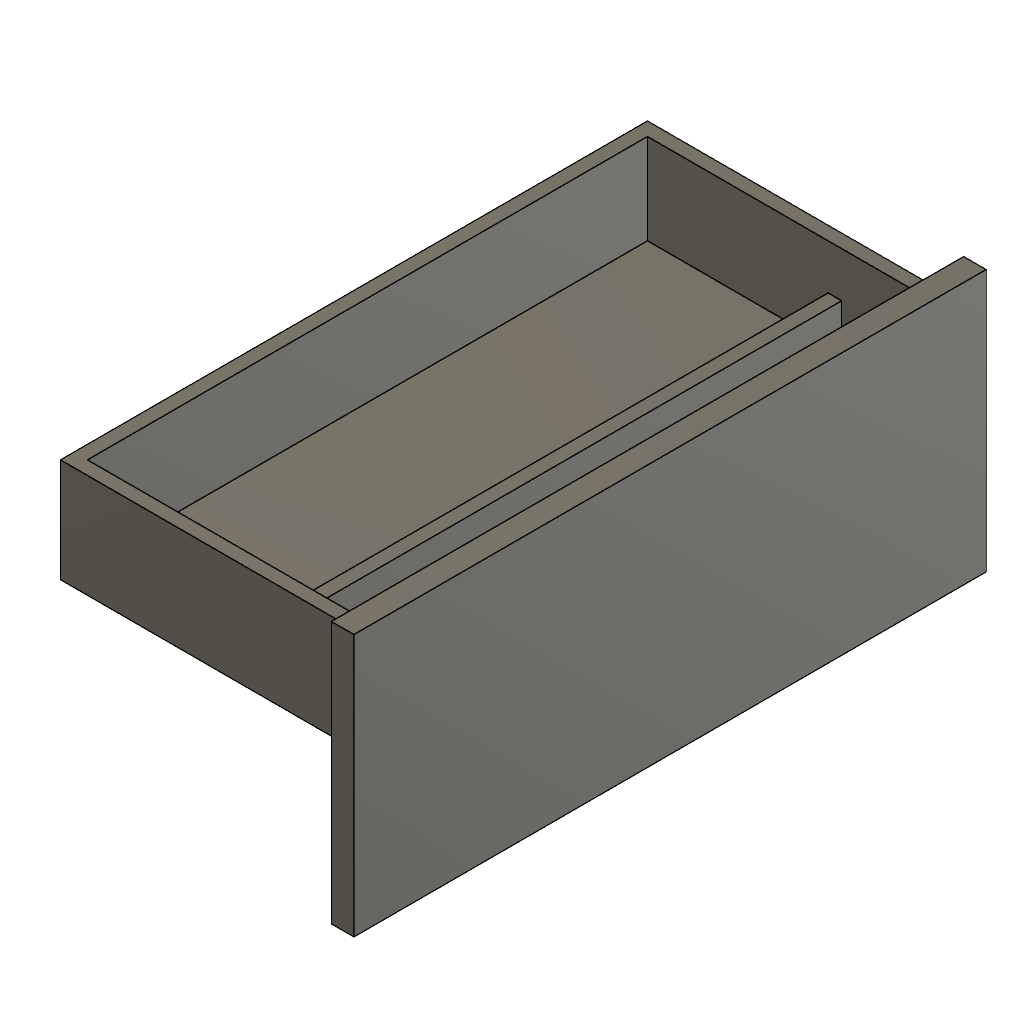
BALANCIN_V2 (Autodesk Fusion 360 archive; units mm, degrees)
design "CAJA BATERIA"
part number: 2026-09-12-01-05-41-271
Autodesk Fusion 360 part; units mm, degrees
sketch "Boceto9" plane through (0, 0, 0) normal (1, 0, 0) x (0, 0, -1)
  line L0 (0, 0) -> (130, 0)
  line L1 (130, 0) -> (130, 3)
  line L2 (130, 3) -> (0, 3)
  line L3 (0, 3) -> (0, 0)
  dimension "d48" = 130
  dimension "d49" = 3
  constraint horizontal L0
  constraint vertical L1
  constraint horizontal L2
  constraint vertical L3
  constraint coincident L0.start L3.end
  measures "d48" distance of L0.start L0.end
  measures "d49" distance of L0.start L2.end
extrude "Extruir9" add sketch "Boceto9" against normal blind 65
sketch "Boceto10" plane through (0, 0, 0) normal (1, 0, 0) x (0, 0, -1)
  line L0 (0, 0) -> (-5, 0)
  line L1 (-5, 0) -> (-5, 27)
  line L2 (-5, 27) -> (135, 27)
  line L3 (135, 27) -> (135, -31)
  line L4 (135, -31) -> (-5, -31)
  line L5 (-5, -31) -> (-5, 27)
  dimension "d64" = 5
  dimension "d65" = 27
  dimension "d66" = 140
  dimension "d67" = 58
  constraint coincident L0.start origin
  constraint horizontal L0
  constraint perpendicular L0 L1
  constraint horizontal L2
  constraint vertical L3
  constraint horizontal L4
  constraint vertical L5
  measures "d64" distance of L0.start L0.end
  measures "d65" distance of L0.end L1.end
  measures "d66" distance of L1.end L2.end
  measures "d67" distance of L1.end L4.end
extrude "Extruir10" add sketch "Boceto10" along normal blind 5
sketch "Boceto11" plane through (0, 3, 0) normal (0, 1, 0) x (-1, 0, 0)
  line L0 (0, 0) -> (0, -130)
  line L1 (0, -130) -> (65, -130)
  line L2 (65, -130) -> (65, 0)
  line L3 (65, 0) -> (0, 0)
  line L4 (0, -130) -> (65, -130)
  line L5 (65, -130) -> (65, -127)
  line L6 (65, -127) -> (0, -127)
  line L7 (0, -127) -> (0, -130)
  line L8 (65, -130) -> (62, -130)
  line L9 (62, -130) -> (62, 0)
  line L10 (62, 0) -> (65, 0)
  line L11 (65, 0) -> (65, -130)
  line L12 (0, 0) -> (65, 0)
  line L13 (65, 0) -> (65, -3)
  line L14 (65, -3) -> (0, -3)
  line L15 (0, -3) -> (0, 0)
  dimension "d59" = 3
  dimension "d60" = 3
  dimension "d61" = 3
  constraint horizontal L4
  constraint vertical L5
  constraint horizontal L6
  constraint vertical L7
  constraint coincident L0.end L1.start
  constraint horizontal L8
  constraint vertical L9
  constraint horizontal L10
  constraint vertical L11
  constraint horizontal L12
  constraint vertical L13
  constraint horizontal L14
  constraint vertical L15
  constraint coincident L0.start L3.end
  measures "d59" distance of L0.end L6.end
  measures "d60" distance of L1.end L8.end
  measures "d61" distance of L0.start L14.end
extrude "Extruir11" add sketch "Boceto11" along normal blind 20 contours L0 L3 L9 L12 L14 L15 | L2 L3 L9 L10 L11 L12 L13 L14 | L0 L1 L4 L6 L7 L9 | L2 L6 L9 L11 L14 | L1 L2 L4 L5 L6 L8 L9 L11
sketch "Boceto12" plane through (0, 3, 0) normal (0, 1, 0) x (-1, 0, 0)
  line L0 (62, -3) -> (0, -3)
  line L1 (0, -3) -> (0, -127)
  line L2 (0, -127) -> (62, -127)
  line L3 (62, -127) -> (62, -3)
  line L4 (62, -127) -> (22, -127)
  line L5 (22, -127) -> (19, -127)
  line L6 (19, -127) -> (19, -7)
  line L7 (19, -7) -> (22, -7)
  line L8 (22, -7) -> (22, -127)
  line L9 (19, -7) -> (39, -7)
  line L10 (39, -7) -> (39, -3)
  line L11 (39, -3) -> (19, -3)
  line L12 (19, -3) -> (19, -7)
  dimension "d68" = 40
  dimension "d69" = 3
  dimension "d70" = 120
  dimension "d71" = 20
  constraint coincident L2.end L3.start
  constraint perpendicular L3 L4
  constraint horizontal L5
  constraint vertical L6
  constraint horizontal L7
  constraint vertical L8
  constraint horizontal L9
  constraint vertical L10
  constraint horizontal L11
  constraint vertical L12
  measures "d68" distance of L2.end L4.end
  measures "d69" distance of L4.end L5.end
  measures "d70" distance of L4.end L7.end
  measures "d71" distance of L6.end L9.end
extrude "Extruir12" add sketch "Boceto12" along normal blind 10 contours L0 L7 L9 L10 L11 L12 | L2 L5 L6 L7 L8 L9

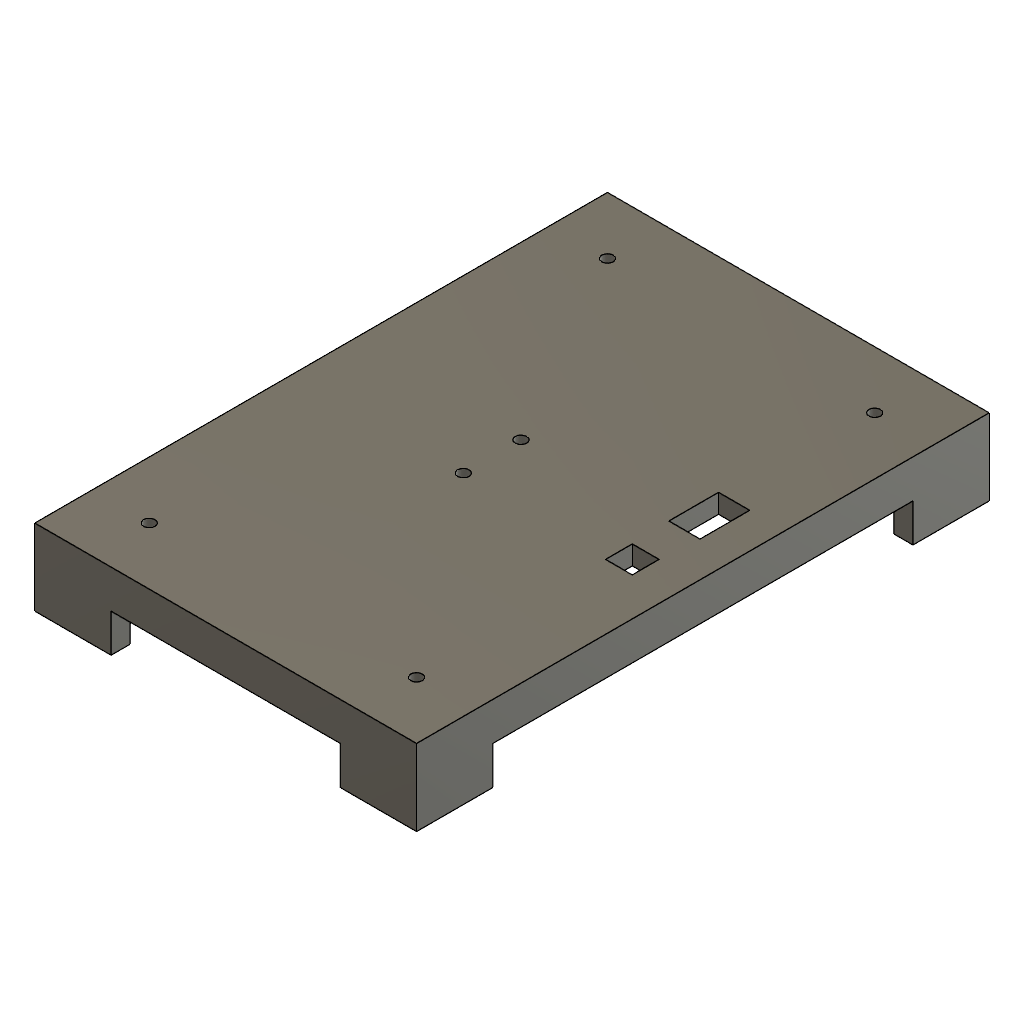
design "TAPA"
part number: 2026-09-12-01-46-28-572
Autodesk Fusion 360 part; units mm, degrees
sketch "Boceto11" plane through (0, 0, 0) normal (0, 1, 0) x (1, 0, 0)
  line L0 (0, 0) -> (100, 0)
  line L1 (100, 0) -> (100, -150)
  line L2 (100, -150) -> (0, -150)
  line L3 (0, -150) -> (0, 0)
  dimension "d80" = 100
  dimension "d81" = 150
  constraint horizontal L0
  constraint vertical L1
  constraint horizontal L2
  constraint vertical L3
  constraint coincident L0.start L3.end
  measures "d80" distance of L0.start L0.end
  measures "d81" distance of L0.start L2.end
extrude "Extruir1" add sketch "Boceto11" along normal blind 5 from surface at 15
sketch "Boceto3" plane through (0, 15, 0) normal (0, -1, 0) x (1, 0, 0)
  line L0 (0, 0) -> (100, 0)
  line L1 (100, 0) -> (100, 5)
  line L2 (100, 5) -> (0, 5)
  line L3 (0, 5) -> (0, 0)
  line L4 (100, 0) -> (95, 0)
  line L5 (95, 0) -> (95, 150)
  line L6 (95, 150) -> (100, 150)
  line L7 (100, 150) -> (100, 0)
  line L8 (100, 150) -> (0, 150)
  line L9 (0, 150) -> (0, 145)
  line L10 (0, 145) -> (100, 145)
  line L11 (100, 145) -> (100, 150)
  line L12 (0, 150) -> (5, 150)
  line L13 (5, 150) -> (5, 0)
  line L14 (5, 0) -> (0, 0)
  line L15 (0, 0) -> (0, 150)
  dimension "d155" = 5
  dimension "d156" = 5
  dimension "d157" = 150
  dimension "d158" = 100
  dimension "d159" = 5
  dimension "d160" = 5
  dimension "d161" = 150
  constraint horizontal L0
  constraint vertical L1
  constraint horizontal L2
  constraint vertical L3
  constraint coincident L0.start L3.end
  constraint horizontal L4
  constraint vertical L5
  constraint horizontal L6
  constraint vertical L7
  constraint horizontal L8
  constraint vertical L9
  constraint horizontal L10
  constraint vertical L11
  constraint horizontal L12
  constraint vertical L13
  constraint horizontal L14
  constraint vertical L15
  measures "d155" distance of L0.start L2.end
  measures "d156" distance of L0.end L4.end
  measures "d157" distance of L0.end L6.end
  measures "d158" distance of L6.end L8.end
  measures "d159" distance of L6.end L10.end
  measures "d160" distance of L8.end L12.end
  measures "d161" distance of L8.end L0.start
extrude "Extruir2" add sketch "Boceto3" along normal blind 15 contours L0 L2 L3 L13 L14 L15 | L0 L2 L5 L13 | L2 L10 L13 L15 | L0 L1 L2 L4 L5 L7 | L8 L9 L10 L12 L13 L15 | L2 L5 L7 L10 | L5 L8 L10 L13 | L5 L6 L7 L8 L10 L11
sketch "Boceto14" plane through (0, 20, 0) normal (0, 1, 0) x (-1, 0, 0)
  line L0 (0, 150) -> (-100, 150)
  line L1 (-100, 150) -> (-100, 0)
  line L2 (-100, 0) -> (0, 0)
  line L3 (0, 0) -> (0, 150)
  line L4 (-100, 150) -> (-100, 80)
  line L5 (-100, 80) -> (-90, 80)
  line L6 (-90, 80) -> (-90, 76.5)
  line L7 (-90, 76.5) -> (-83, 76.5)
  line L8 (-83, 76.5) -> (-83, 83.5)
  line L9 (-83, 83.5) -> (-90, 83.5)
  line L10 (-90, 83.5) -> (-90, 76.5)
  line L11 (-86.5, 76.5) -> (-86.5, 66.5)
  line L12 (-86.5, 66.5) -> (-100, 66.5)
  line L13 (-86.5, 66.5) -> (-82.5879, 66.5)
  line L14 (-82.5879, 66.5) -> (-90.7379, 66.5)
  line L15 (-90.7379, 66.5) -> (-90.7379, 53.5)
  line L16 (-90.7379, 53.5) -> (-82.5879, 53.5)
  line L17 (-82.5879, 53.5) -> (-82.5879, 66.5)
  dimension "d106" = 70
  dimension "d107" = 10
  dimension "d108" = 3.5
  dimension "d109" = 7
  dimension "d110" = 7
  dimension "d122" = 10
  dimension "d123" = 8.15
  dimension "d124" = 13
  constraint coincident L0.end L1.start
  constraint perpendicular L0 L4
  constraint perpendicular L4 L5
  constraint perpendicular L5 L6
  constraint horizontal L7
  constraint vertical L8
  constraint horizontal L9
  constraint vertical L10
  constraint midpoint L7 L11.start
  constraint perpendicular L7 L11
  constraint coincident L1 L12.end
  constraint perpendicular L1 L12
  constraint perpendicular L11 L13
  constraint horizontal L14
  constraint vertical L15
  constraint horizontal L16
  constraint vertical L17
  measures "d106" distance of L0.end L4.end
  measures "d107" distance of L4.end L5.end
  measures "d108" distance of L5.end L6.end
  measures "d109" distance of L6.end L7.end
  measures "d110" distance of L6.end L9.end
  measures "d122" distance of L11.start L11.end
  measures "d123" distance of L13.end L14.end
  measures "d124" distance of L13.end L16.end
extrude "Extruir9" cut sketch "Boceto14" against normal blind 30 contours L6 L7 L8 L9 L10 | L12 L13 L14 L15 L16 L17
sketch "Boceto15" plane through (0, 0, 150) normal (0, 0, 1) x (1, 0, 0)
  line L0 (100, 0) -> (100, 20)
  line L1 (100, 20) -> (0, 20)
  line L2 (0, 20) -> (0, 0)
  line L3 (0, 0) -> (100, 0)
  line L4 (0, 0) -> (20, 0)
  line L5 (100, 0) -> (80, 0)
  line L6 (80, 0) -> (20, 0)
  line L7 (20, 0) -> (20, 10)
  line L8 (20, 10) -> (80, 10)
  line L9 (80, 10) -> (80, 0)
  dimension "d113" = 20
  dimension "d114" = 20
  dimension "d115" = 10
  constraint coincident L2.end L3.start
  constraint perpendicular L2 L4
  constraint coincident L0.start L3.end
  constraint perpendicular L0 L5
  constraint horizontal L6
  constraint vertical L7
  constraint horizontal L8
  constraint vertical L9
  measures "d113" distance of L2.end L4.end
  measures "d114" distance of L0.start L5.end
  measures "d115" distance of L5.end L8.end
extrude "Extruir10" cut sketch "Boceto15" against normal blind 180 contours L3 L6 L7 L8 L9
sketch "Boceto16" plane through (100, 0, 0) normal (1, 0, 0) x (0, 0, -1)
  line L0 (0, 0) -> (0, 20)
  line L1 (0, 20) -> (-150, 20)
  line L2 (-150, 20) -> (-150, 0)
  line L3 (-150, 0) -> (0, 0)
  line L4 (0, 0) -> (-20, 0)
  line L5 (-150, 0) -> (-130, 0)
  line L6 (-130, 0) -> (-20, 0)
  line L7 (-20, 0) -> (-20, 10)
  line L8 (-20, 10) -> (-130, 10)
  line L9 (-130, 10) -> (-130, 0)
  dimension "d118" = 20
  dimension "d119" = 20
  constraint coincident L0.start L3.end
  constraint perpendicular L0 L4
  constraint coincident L2.end L3.start
  constraint perpendicular L2 L5
  constraint horizontal L6
  constraint vertical L7
  constraint horizontal L8
  constraint vertical L9
  measures "d118" distance of L0.start L4.end
  measures "d119" distance of L2.end L5.end
extrude "Extruir11" cut sketch "Boceto16" against normal blind 130 contours L3 L6 L7 L8 L9
sketch "Boceto17" plane through (0, 20, 0) normal (0, 1, 0) x (-1, 0, 0)
  line L0 (-83, 76.5) -> (-90, 76.5)
  line L1 (-90, 76.5) -> (-90, 83.5)
  line L2 (-90, 83.5) -> (-83, 83.5)
  line L3 (-83, 83.5) -> (-83, 76.5)
  line L4 (-90.7379, 66.5) -> (-82.5879, 66.5)
  line L5 (-82.5879, 66.5) -> (-82.5879, 53.5)
  line L6 (-82.5879, 53.5) -> (-90.7379, 53.5)
  line L7 (-90.7379, 53.5) -> (-90.7379, 66.5)
  line L8 (0, 150) -> (-100, 150)
  line L9 (-100, 150) -> (-100, 0)
  line L10 (-100, 0) -> (0, 0)
  line L11 (0, 0) -> (0, 150)
  line L12 (-100, 0) -> (-85, 0)
  line L13 (-85, 0) -> (-85, 15)
  circle A0 centre (-85, 15) radius 1.5
  line L14 (0, 0) -> (-15, 0)
  line L15 (-15, 0) -> (-15, 15)
  circle A1 centre (-15, 15) radius 1.5
  line L16 (0, 150) -> (-15, 150)
  line L17 (-15, 150) -> (-15, 135)
  circle A2 centre (-15, 135) radius 1.5
  line L18 (-100, 150) -> (-85, 150)
  line L19 (-85, 150) -> (-85, 135)
  circle A3 centre (-85, 135) radius 1.5
  dimension "d125" = 15
  dimension "d126" = 15
  dimension "d127" = 3
  dimension "d128" = 15
  dimension "d129" = 15
  dimension "d130" = 3
  dimension "d131" = 15
  dimension "d132" = 15
  dimension "d133" = 3
  dimension "d134" = 15
  dimension "d135" = 15
  dimension "d136" = 3
  constraint coincident L9.end L10.start
  constraint perpendicular L9 L12
  constraint perpendicular L10 L13
  constraint coincident L13.end A0.centre
  constraint coincident L10.end L11.start
  constraint perpendicular L11 L14
  constraint perpendicular L10 L15
  constraint coincident L15.end A1.centre
  constraint coincident L8.start L11.end
  constraint perpendicular L11 L16
  constraint perpendicular L8 L17
  constraint coincident L17.end A2.centre
  constraint coincident L8.end L9.start
  constraint perpendicular L9 L18
  constraint perpendicular L8 L19
  constraint coincident L19.end A3.centre
  measures "d125" distance of L9.end L12.end
  measures "d126" distance of L12.end L13.end
  measures "d127" diameter of A0
  measures "d128" distance of L10.end L14.end
  measures "d129" distance of L14.end L15.end
  measures "d130" diameter of A1
  measures "d131" distance of L8.start L16.end
  measures "d132" distance of L16.end L17.end
  measures "d133" diameter of A2
  measures "d134" distance of L8.end L18.end
  measures "d135" distance of L18.end L19.end
  measures "d136" diameter of A3
extrude "Extruir12" cut sketch "Boceto17" against normal blind 20 contours A0 | A1 | A2 | A3
sketch "Boceto18" plane through (0, 15, 0) normal (0, -1, 0) x (1, 0, 0)
  line L0 (95, 140) -> (95, 10)
  line L1 (95, 140) -> (95, 75)
  line L2 (95, 75) -> (50, 75)
  line L3 (50, 75) -> (50, 85.35)
  line L4 (50, 85.35) -> (42, 85.35)
  line L5 (42, 85.35) -> (58, 85.35)
  line L6 (58, 85.35) -> (58, 64.65)
  line L7 (58, 64.65) -> (42, 64.65)
  line L8 (42, 64.65) -> (42, 85.35)
  line L9 (95, 145) -> (5, 145)
  line L10 (5, 145) -> (5, 5)
  line L11 (5, 5) -> (95, 5)
  line L12 (95, 5) -> (95, 145)
  line L13 (82.5879, 66.5) -> (90.7379, 66.5)
  line L14 (90.7379, 66.5) -> (90.7379, 53.5)
  line L15 (90.7379, 53.5) -> (82.5879, 53.5)
  line L16 (82.5879, 53.5) -> (82.5879, 66.5)
  line L17 (90, 76.5) -> (83, 76.5)
  line L18 (83, 76.5) -> (83, 83.5)
  line L19 (83, 83.5) -> (90, 83.5)
  line L20 (90, 83.5) -> (90, 76.5)
  circle A0 centre (15, 135) radius 1.5
  circle A1 centre (15, 15) radius 1.5
  circle A2 centre (85, 135) radius 1.5
  circle A3 centre (85, 15) radius 1.5
  line L21 (100, 0) -> (0, 0)
  dimension "d140" = 45
  dimension "d141" = 10.35
  dimension "d142" = 8
  dimension "d143" = 16
  dimension "d144" = 20.7
  dimension "d162" = 75
  constraint midpoint L0 L1.end
  constraint perpendicular L2 L3
  constraint perpendicular L3 L4
  constraint horizontal L5
  constraint vertical L6
  constraint horizontal L7
  constraint vertical L8
  measures "d140" distance of L1.end L2.end
  measures "d141" distance of L2.end L3.end
  measures "d142" distance of L3.end L4.end
  measures "d143" distance of L4.end L5.end
  measures "d144" distance of L4.end L7.end
  measures "d162" distance of L2 L21
extrude "Extruir13" cut sketch "Boceto18" against normal blind 2 contours L2 L3 L4 L5 L6 L7 L8 | L2 L3 L5 L6
sketch "Boceto19" plane through (0, 17, 0) normal (0, -1, 0) x (1, 0, 0)
  line L0 (42, 64.65) -> (58, 64.65)
  line L1 (58, 64.65) -> (58, 85.35)
  line L2 (58, 85.35) -> (42, 85.35)
  line L3 (42, 85.35) -> (42, 64.65)
  line L4 (42, 64.65) -> (44.8, 64.65)
  line L5 (44.8, 64.65) -> (44.8, 67.45)
  line L6 (44.8, 67.45) -> (42, 67.45)
  line L7 (42, 67.45) -> (42, 64.65)
  line L8 (42, 85.35) -> (44.8, 85.35)
  line L9 (44.8, 85.35) -> (44.8, 82.55)
  line L10 (44.8, 82.55) -> (42, 82.55)
  line L11 (42, 82.55) -> (42, 85.35)
  circle A0 centre (44.8, 82.55) radius 1.5
  circle A1 centre (44.8, 67.45) radius 1.5
  dimension "d147" = 2.8
  dimension "d148" = 2.8
  dimension "d149" = 2.8
  dimension "d150" = 2.8
  dimension "d163" = 20.7
  dimension "d164" = 16
  dimension "d165" = 3
  dimension "d166" = 3
  constraint horizontal L4
  constraint vertical L5
  constraint horizontal L6
  constraint vertical L7
  constraint coincident L0.start L3.end
  constraint horizontal L8
  constraint vertical L9
  constraint horizontal L10
  constraint vertical L11
  constraint coincident L2.end L3.start
  constraint coincident L9.end L10.start
  constraint coincident L5.end L6.start
  measures "d147" distance of L0.start L4.end
  measures "d148" distance of L0.start L6.end
  measures "d149" distance of L2.end L8.end
  measures "d150" distance of L2.end L10.end
  measures "d163" distance of L0 L2
  measures "d164" distance of L1 L3
  measures "d165" diameter of A0
  measures "d166" diameter of A1
extrude "Extruir14" cut sketch "Boceto19" against normal blind 3.5 contours L5 L6 A1 | L5 L6 A1 | L9 L10 A0 | L9 L10 A0

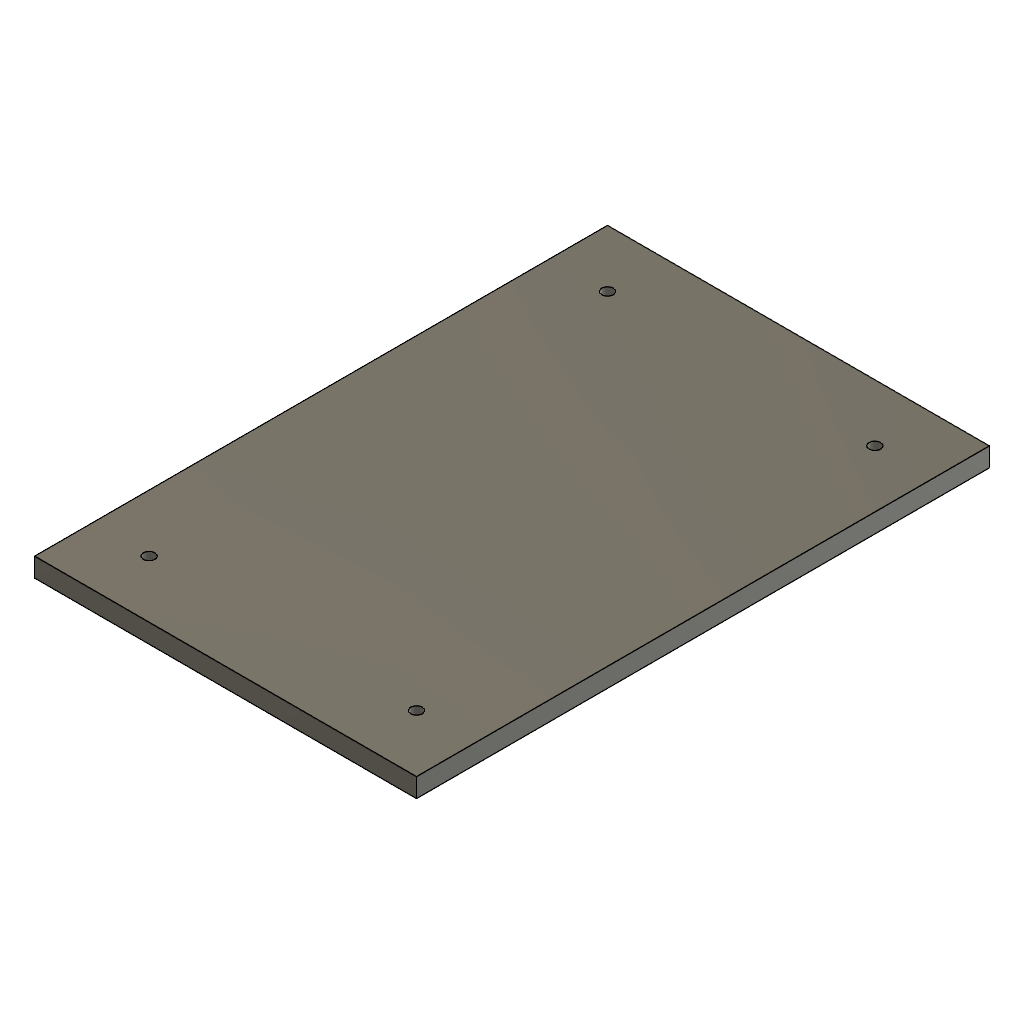
design "PLACA"
part number: 2026-09-12-02-16-54-781
Autodesk Fusion 360 part; units mm, degrees
sketch "Boceto1" plane through (2.5309, 197.6555, 0.0134) normal (0, 1, 0) x (-1, 0, 0)
  line L0 (0, 0) -> (-100, 0)
  line L1 (-100, 0) -> (-100, 150)
  line L2 (-100, 150) -> (0, 150)
  line L3 (0, 150) -> (0, 0)
  line L4 (-100, 150) -> (-85, 150)
  line L5 (-85, 150) -> (-85, 135)
  line L6 (0, 150) -> (-15, 150)
  line L7 (-15, 150) -> (-15, 135)
  line L8 (-100, 0) -> (-85, 0)
  line L9 (-85, 0) -> (-85, 15)
  line L10 (0, 0) -> (-15, 0)
  line L11 (-15, 0) -> (-15, 15)
  circle A0 centre (-15, 15) radius 1.5
  circle A1 centre (-85, 15) radius 1.5
  circle A2 centre (-15, 135) radius 1.5
  circle A3 centre (-85, 135) radius 1.5
  dimension "d3" = 100
  dimension "d4" = 150
  dimension "d5" = 15
  dimension "d6" = 15
  dimension "d7" = 15
  dimension "d8" = 15
  dimension "d9" = 15
  dimension "d10" = 15
  dimension "d11" = 15
  dimension "d12" = 3
  dimension "d13" = 3
  dimension "d14" = 3
  dimension "d15" = 3
  dimension "d16" = 15
  constraint horizontal L0
  constraint vertical L1
  constraint horizontal L2
  constraint vertical L3
  constraint coincident L0.start L3.end
  constraint perpendicular L1 L4
  constraint perpendicular L2 L5
  constraint perpendicular L3 L6
  constraint perpendicular L2 L7
  constraint perpendicular L1 L8
  constraint perpendicular L8 L9
  constraint coincident L0 L10.end
  constraint perpendicular L0 L11
  constraint coincident L11.end A0.centre
  constraint coincident L9.end A1.centre
  constraint coincident L7.end A2.centre
  constraint coincident L5.end A3.centre
  measures "d3" distance of L0.start L0.end
  measures "d4" distance of L0.start L2.end
  measures "d5" distance of L1.end L4.end
  measures "d6" distance of L4.end L5.end
  measures "d7" distance of L2.end L6.end
  measures "d8" distance of L6.end L7.end
  measures "d9" distance of L0.end L8.end
  measures "d10" distance of L8.end L9.end
  measures "d11" distance of L0.start L10.end
  measures "d12" diameter of A0
  measures "d13" diameter of A1
  measures "d14" diameter of A2
  measures "d15" diameter of A3
  measures "d16" distance of L10.end L11.end
extrude "Extruir1" add sketch "Boceto1" along normal blind 5

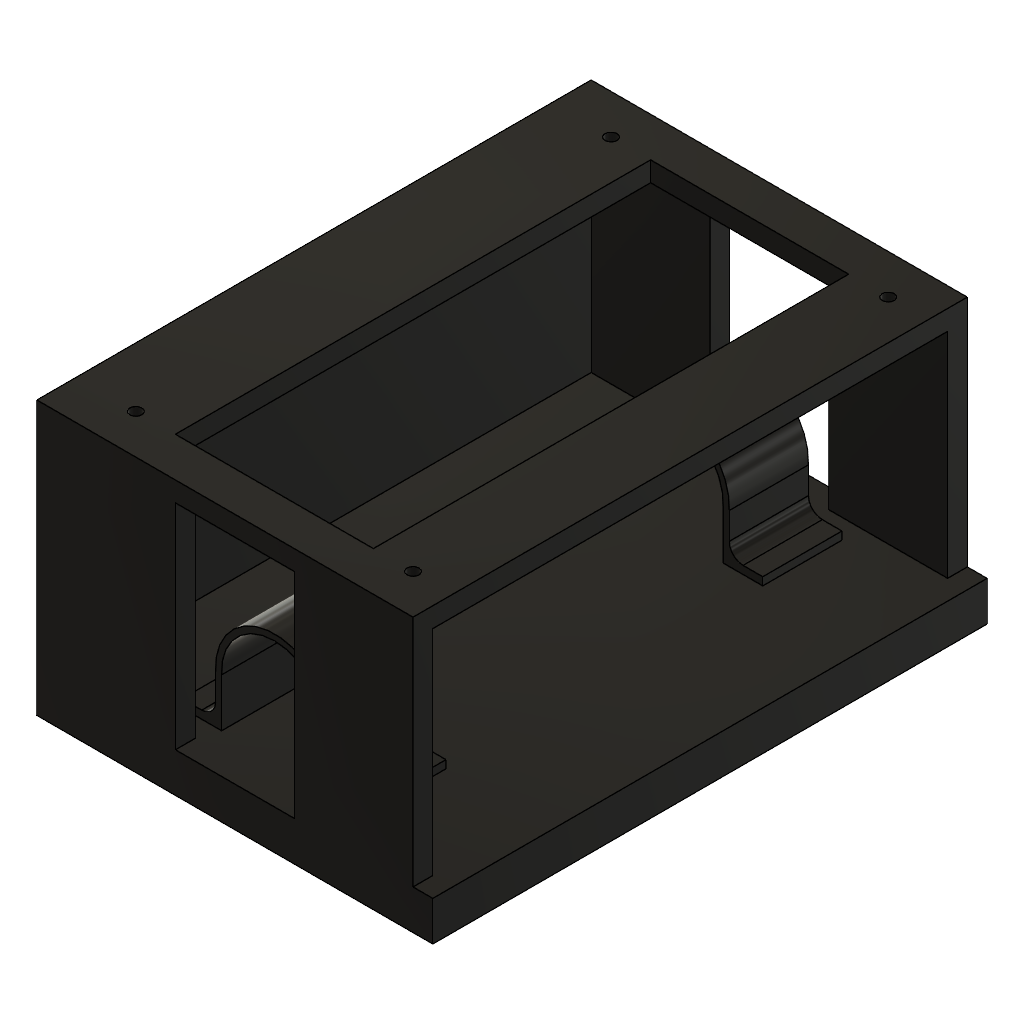
design "BASE"
part number: 2026-09-12-00-28-25-812
Autodesk Fusion 360 part; units mm, degrees
other "DerivedContext1"
sketch "Boceto3" plane through (0, 0, 0) normal (1, 0, 0) x (0, 0, -1)
  line L0 (0, 0) -> (0, 20)
  line L1 (0, 20) -> (-70, 20)
  line L2 (0, 20) -> (70, 20)
  line L3 (-70, 20) -> (70, 20)
  line L4 (70, 20) -> (70, 10)
  line L5 (70, 10) -> (-70, 10)
  line L6 (-70, 10) -> (-70, 20)
  dimension "d3" = 10
  dimension "d17" = 20
  dimension "d75" = 70
  dimension "d76" = 70
  constraint coincident L0.start origin
  constraint perpendicular L0 L1
  constraint perpendicular L0 L2
  constraint horizontal L3
  constraint vertical L4
  constraint horizontal L5
  constraint vertical L6
  measures "d3" distance of L1.end L5.end
  measures "d17" distance of L0.start L0.end
  measures "d75" distance of L0 L4
  measures "d76" distance of L0 L6
extrude "Extruir1" add sketch "Boceto3" along normal mid plane 100
sketch "Boceto4" plane through (0, 20, 0) normal (0, 1, 0) x (-1, 0, 0)
  line L0 (-50, 70) -> (50, 70)
  line L1 (50, 70) -> (50, 65)
  line L2 (50, 65) -> (-50, 65)
  line L3 (-50, 65) -> (-50, 70)
  line L4 (50, -70) -> (-50, -70)
  line L5 (-50, -70) -> (-50, -65)
  line L6 (-50, -65) -> (50, -65)
  line L7 (50, -65) -> (50, -70)
  line L8 (50, 70) -> (45, 70)
  line L9 (45, 70) -> (45, -70)
  line L10 (45, -70) -> (50, -70)
  line L11 (50, -70) -> (50, 70)
  line L12 (-50, 70) -> (0, 70)
  line L13 (0, 70) -> (-15, 70)
  line L14 (-15, 70) -> (-15, 65)
  line L15 (-15, 65) -> (0, 65)
  line L16 (0, 70) -> (15, 70)
  line L17 (15, 70) -> (15, 65)
  line L18 (15, 65) -> (0, 65)
  line L19 (0, -65) -> (-15, -65)
  line L20 (-15, -65) -> (-15, -70)
  line L21 (-15, -70) -> (0, -70)
  line L22 (0, -65) -> (15, -65)
  line L23 (15, -65) -> (15, -70)
  line L24 (15, -70) -> (0, -70)
  line L25 (-50, -70) -> (-45, -70)
  line L26 (-45, -70) -> (-45, -65)
  line L27 (-45, -65) -> (-50, -65)
  line L28 (-50, -65) -> (-50, -70)
  line L29 (-50, 70) -> (-45, 70)
  line L30 (-45, 70) -> (-45, 65)
  line L31 (-45, 65) -> (-50, 65)
  line L32 (-50, 65) -> (-50, 70)
  dimension "d77" = 100
  dimension "d78" = 5
  dimension "d83" = 15
  dimension "d84" = 15
  dimension "d85" = 15
  dimension "d86" = 5
  dimension "d87" = 15
  dimension "d88" = 5
  dimension "d97" = 5
  dimension "d98" = 5
  dimension "d99" = 5
  constraint horizontal L0
  constraint vertical L1
  constraint horizontal L2
  constraint vertical L3
  constraint horizontal L4
  constraint vertical L5
  constraint horizontal L6
  constraint vertical L7
  constraint horizontal L8
  constraint vertical L9
  constraint horizontal L10
  constraint vertical L11
  constraint coincident L4 L9.end
  constraint midpoint L0 L12.end
  constraint horizontal L13
  constraint vertical L14
  constraint horizontal L15
  constraint horizontal L16
  constraint vertical L17
  constraint horizontal L18
  constraint horizontal L19
  constraint vertical L20
  constraint horizontal L21
  constraint midpoint L6 L19.start
  constraint horizontal L22
  constraint vertical L23
  constraint horizontal L24
  constraint horizontal L25
  constraint vertical L26
  constraint horizontal L27
  constraint vertical L28
  constraint horizontal L29
  constraint vertical L30
  constraint horizontal L31
  constraint vertical L32
  measures "d77" distance of L0.start L0.end
  measures "d78" distance of L0.start L2.end
  measures "d83" distance of L12.end L13.end
  measures "d84" distance of L12.end L16.end
  measures "d85" distance of L19.start L19.end
  measures "d86" distance of L19.start L21.end
  measures "d87" distance of L19.start L22.end
  measures "d88" distance of L19.start L21.end
  measures "d97" distance of L4.end L25.end
  measures "d98" distance of L0.start L29.end
  measures "d99" distance of L0.start L2.end
extrude "Extruir2" add sketch "Boceto4" along normal blind 54 contours L0 L2 L12 L14 L30 | L0 L2 L9 L17 | L0 L1 L2 L8 L9 L11 | L2 L6 L9 L11 | L4 L6 L9 L23 | L4 L6 L7 L9 L10 L11 | L4 L6 L20 L26
sketch "Boceto6" plane through (0, 74, 0) normal (0, 1, 0) x (-1, 0, 0)
  line L0 (50, -70) -> (25, -70)
  line L1 (25, -70) -> (25, 70)
  line L2 (25, 70) -> (50, 70)
  line L3 (50, 70) -> (50, -70)
  line L4 (25, -70) -> (-25, -70)
  line L5 (-25, -70) -> (-25, -60)
  line L6 (-25, -60) -> (25, -60)
  line L7 (25, -60) -> (25, -70)
  line L8 (-50, -70) -> (-25, -70)
  line L9 (-25, -70) -> (-25, 70)
  line L10 (25, 60) -> (25, 70)
  line L11 (25, 70) -> (-25, 70)
  line L12 (-25, 70) -> (-25, 60)
  line L13 (-25, 60) -> (25, 60)
  line L14 (25, 60) -> (25, 70)
  line L15 (-45, -70) -> (-25, -70)
  line L16 (-25, -70) -> (-25, 70)
  line L17 (-25, 70) -> (-45, 70)
  line L18 (-45, 70) -> (-45, -70)
  dimension "d89" = 25
  dimension "d90" = 50
  dimension "d91" = 10
  dimension "d95" = 25
  dimension "d96" = 10
  constraint horizontal L0
  constraint vertical L1
  constraint horizontal L2
  constraint vertical L3
  constraint horizontal L4
  constraint vertical L5
  constraint horizontal L6
  constraint vertical L7
  constraint horizontal L8
  constraint vertical L9
  constraint vertical L10
  constraint horizontal L11
  constraint vertical L12
  constraint horizontal L13
  constraint vertical L14
  constraint horizontal L15
  constraint vertical L16
  constraint horizontal L17
  constraint vertical L18
  constraint coincident L8 L15.start
  measures "d89" distance of L0.start L0.end
  measures "d90" distance of L0.end L4.end
  measures "d91" distance of L0.end L6.end
  measures "d95" distance of L8.start L4.end
  measures "d96" distance of L1.end L10.start
extrude "Extruir4" add sketch "Boceto6" 1 faces at (-48.3333, 74, -21.6667) along normal blind 5 contours L0 L1 L2 L3 L7 L10 L14 | L1 L4 L5 L6 L7 L9 L16 | L5 L8 L9 L12 L15 L16 L17 L18 | L1 L9 L10 L11 L12 L13 L14 L16
sketch "Boceto8" plane through (0, 0, 0) normal (0, 0, 1) x (1, 0, 0)
  circle A0 centre (0, 33) radius 13.3417
  circle A1 centre (0, 33) radius 14.8661
  line L0 (-14.8465, 32.2379) -> (-14.8465, 25.5)
  line L1 (-13.3199, 32.2379) -> (-13.3199, 20)
  line L2 (14.8465, 32.2379) -> (14.8465, 25.5)
  line L3 (13.3199, 32.2379) -> (13.3199, 20)
  line L4 (13.3199, 20) -> (14.8465, 20)
  line L5 (-14.8465, 20) -> (-13.3199, 20)
  line L6 (-13.3199, 20) -> (-23.3199, 20)
  line L7 (-23.3199, 20) -> (-23.3199, 22)
  line L8 (-23.3199, 22) -> (-18.3465, 22)
  line L9 (-13.3199, 22) -> (-13.3199, 20)
  arc A2 (-18.3465, 22) -> (-14.8465, 25.5) centre (-18.3465, 25.5) ccw
  line L10 (13.3199, 20) -> (23.3199, 20)
  line L11 (23.3199, 20) -> (23.3199, 22)
  line L12 (23.3199, 22) -> (18.3465, 22)
  line L13 (13.3199, 22) -> (13.3199, 20)
  arc A3 (14.8465, 25.5) -> (18.3465, 22) centre (18.3465, 25.5) ccw
  dimension "d42" = 10
  dimension "d43" = 2
  dimension "d44" = 3.5
  dimension "d45" = 10
  dimension "d46" = 2
  dimension "d47" = 3.5
  constraint concentric A0 A1
  constraint coincident A1 L0.start
  constraint vertical L0
  constraint coincident A0 L1.start
  constraint vertical L1
  constraint coincident A1 L2.start
  constraint parallel L1 L2
  constraint coincident A0 L3.start
  constraint parallel L2 L3
  constraint perpendicular L2 L4
  constraint perpendicular L0 L5
  constraint horizontal L6
  constraint vertical L7
  constraint horizontal L8
  constraint vertical L9
  constraint coincident L9.start L8
  constraint coincident L5.start L0
  constraint tangent L8 A2
  constraint tangent L0 A2
  constraint horizontal L10
  constraint vertical L11
  constraint horizontal L12
  constraint vertical L13
  constraint coincident L13.start L12
  constraint coincident L4.end L2
  constraint tangent L12 A3
  constraint tangent L2 A3
  measures "d42" distance of L1.end L6.end
  measures "d43" distance of L1.end L9.start
  measures "d44" radius of A2
  measures "d45" distance of L3.end L10.end
  measures "d46" distance of L3.end L13.start
  measures "d47" radius of A3
extrude "Extruir6" add sketch "Boceto8" along normal blind 20 from surface at 40 contours A0 A1 L1 L3 | A1 L0 L1 L5 L6 L7 L8 L9 A2 | A1 L2 L3 L4 L10 L11 L12 L13 A3 picked at (-14.3123, 33.6022)
extrude "Extruir7" add sketch "Boceto8" along normal blind 20 from surface at -60 contours A0 A1 L1 L3 | A1 L0 L1 L5 L6 L7 L8 L9 A2 | A1 L2 L3 L4 L10 L11 L12 L13 A3 picked at (-14.3123, 33.6022)
sketch "Boceto13" plane through (0, 79, 0) normal (0, 1, 0) x (-1, 0, 0)
  line L0 (-45, -70) -> (50, -70)
  line L1 (50, -70) -> (50, 70)
  line L2 (50, 70) -> (-45, 70)
  line L3 (-45, 70) -> (-45, -70)
  line L4 (-25, -60) -> (-25, 60)
  line L5 (-25, 60) -> (25, 60)
  line L6 (25, 60) -> (25, -60)
  line L7 (25, -60) -> (-25, -60)
  line L8 (50, -70) -> (35, -70)
  line L9 (35, -70) -> (35, -60)
  circle A0 centre (35, -60) radius 1.5
  line L10 (-45, -70) -> (-35, -70)
  line L11 (-35, -70) -> (-35, -60)
  circle A1 centre (-35, -60) radius 1.5
  line L12 (50, 70) -> (35, 70)
  line L13 (35, 70) -> (35, 60)
  circle A2 centre (35, 60) radius 1.5
  line L14 (-45, 70) -> (-35, 70)
  line L15 (-35, 70) -> (-35, 60)
  circle A3 centre (-35, 60) radius 1.5
  dimension "d100" = 15
  dimension "d101" = 10
  dimension "d102" = 3
  dimension "d103" = 10
  dimension "d104" = 10
  dimension "d105" = 3
  dimension "d106" = 15
  dimension "d107" = 10
  dimension "d108" = 3
  dimension "d109" = 10
  dimension "d110" = 10
  dimension "d111" = 3
  constraint coincident L0.end L1.start
  constraint perpendicular L1 L8
  constraint perpendicular L8 L9
  constraint coincident L9.end A0.centre
  constraint coincident L0.start L3.end
  constraint perpendicular L3 L10
  constraint perpendicular L10 L11
  constraint coincident L11.end A1.centre
  constraint coincident L1.end L2.start
  constraint perpendicular L6 L12
  constraint perpendicular L2 L13
  constraint coincident L13.end A2.centre
  constraint coincident L2.end L3.start
  constraint perpendicular L3 L14
  constraint perpendicular L14 L15
  constraint coincident L15.end A3.centre
  measures "d100" distance of L0.end L8.end
  measures "d101" distance of L8.end L9.end
  measures "d102" diameter of A0
  measures "d103" distance of L0.start L10.end
  measures "d104" distance of L10.end L11.end
  measures "d105" diameter of A1
  measures "d106" distance of L1.end L12.end
  measures "d107" distance of L12.end L13.end
  measures "d108" diameter of A2
  measures "d109" distance of L2.end L14.end
  measures "d110" distance of L14.end L15.end
  measures "d111" diameter of A3
extrude "Extruir13" cut sketch "Boceto13" against normal blind 7 contours A0 | A1 | A2 | A3

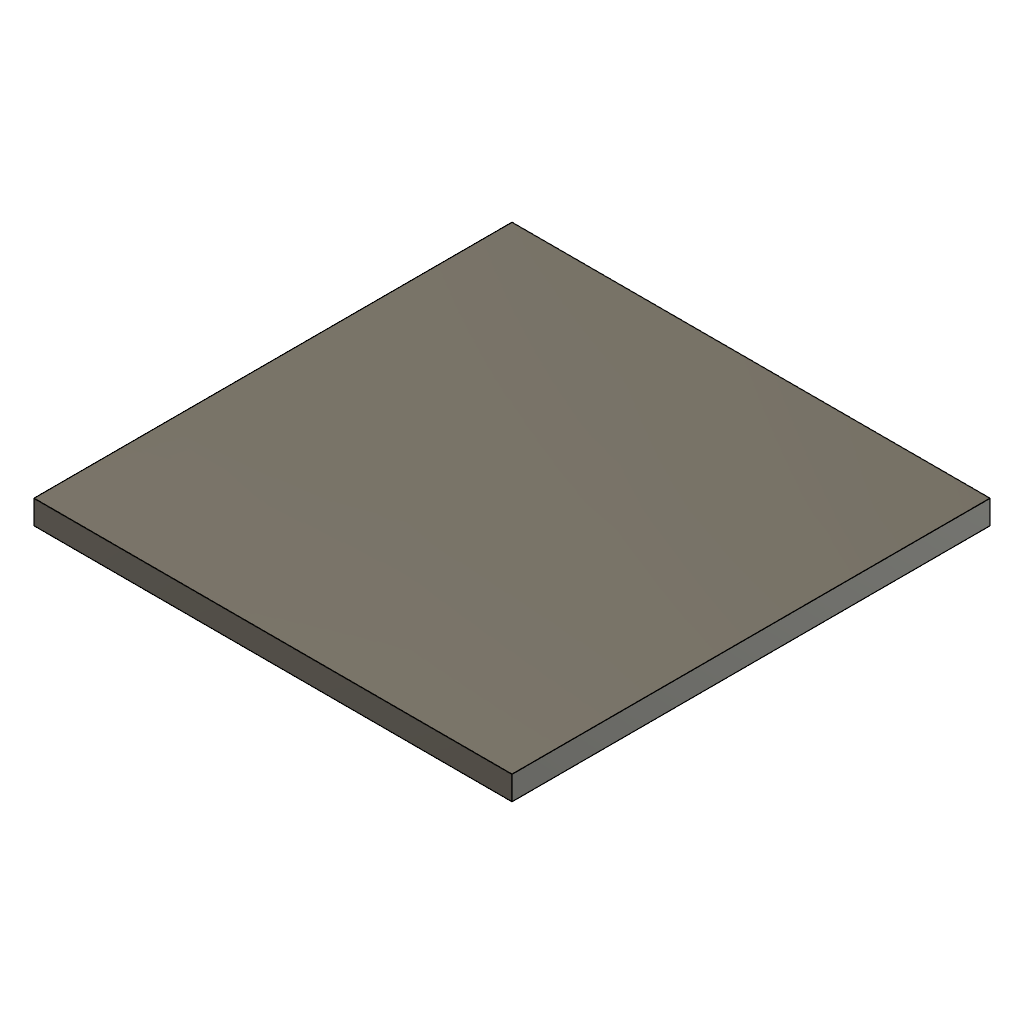
design "SUELO"
part number: 2026-09-16-12-44-53-559
Autodesk Fusion 360 part; units mm, degrees
sketch "Boceto1" plane through (0, 0, 0) normal (0, 1, 0) x (1, 0, 0)
  line L0 (100, 100) -> (-100, 100)
  line L1 (-100, 100) -> (-100, -100)
  line L2 (-100, -100) -> (100, -100)
  line L3 (100, -100) -> (100, 100)
  constraint horizontal L0
  constraint vertical L1
  constraint horizontal L2
  constraint vertical L3
extrude "Extruir1" add sketch "Boceto1" against normal blind 10
